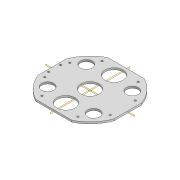
# Autodesk Inventor part: Drone_plate_3
Saved by Autodesk Inventor 2022 (Build 260153000, 153)
## iProperties
Created: 2022-04-28
Part Number: Drone_plate_3
Material: Generic
Document SubType Name: Modeling
Designer: dell
Density: 1 g/cm^3
Appearance: Default
Mass: 28.3386 g
Surface Area: 222.49 cm^2
Volume: 28.3386 cm^3
Author: dell
Autodesk Inventor part; units mm, degrees
ref_plane "XZ Plane" through (0, 0, 0) normal (0, 1, 0) x (-1, 0, 0)
ref_plane "XY Plane" through (0, 0, 0) normal (0, 0, 1) x (1, 0, 0)
sketch "Sketch1" plane through (0, 0, 0) normal (0, 1, 0) x (-1, 0, 0)
  line L0 (0, 0) -> (60, 0)
  line L1 (60, 0) -> (60, -120)
  line L2 (60, -120) -> (0, -120)
  line L3 (0, -120) -> (0, 0)
  line L4 (60, 0) -> (0, -120) construction
  line L5 (60, -120) -> (0, 0) construction
  circle A0 centre (30, -60) radius 67.082
  line L6 (30, -120) -> (30, 7.082) construction
  line L7 (60, -60) -> (0, -60)
  line L8 (30, -60) -> (81.3878, -103.1195) construction
  line L9 (41.76, -45.985) -> (17.4815, -74.919) construction
  line L10 (-33, -36.9566) -> (-33, -83.0434)
  line L11 (93, -36.9566) -> (93, -83.0434)
  circle A1 centre (60, -110) radius 1.5
  circle A2 centre (70, -60) radius 12.5
  circle A3 centre (30, -100) radius 15
  circle A4 centre (84.4498, -80.8618) radius 1.5
  circle A5 centre (68.3022, -92.1394) radius 10
  circle A6 centre (30, -60) radius 15
  point P0 (60, -120)
  point P1 (60, 0)
  dimension "d0" = 120
  dimension "d25" = 60
  dimension "d27" = 50
  dimension "d38" = 63
  dimension "d39" = 63
  dimension "d50" = 3
  dimension "d51" = 10
  dimension "d52" = 25
  dimension "d53" = 40
  dimension "d54" = 30
  dimension "d55" = 40
  dimension "d56" = 20
  dimension "d57" = 50
  dimension "d58" = 30
  constraints: 24 end point, 6 centre point, 6 midpoint, 4 point on line, 3 parallel, 3 perpendicular, 2 coincident, 1 horizontal, 1 horizontal alignment, 1 symmetric about line, 1 vertical, 10 other
  measures "d0" distance of L2.end L0.start
  measures "d25" distance between parallel lines of L1 L3
  measures "d27" angle of L6 L8
  measures "d38" distance from line of point (30, -60) L10
  measures "d39" distance from line of point (30, -60) L11
  measures "d50" diameter of A1
  measures "d51" distance of L1.end A1.centre
  measures "d52" diameter of A2
  measures "d53" distance of L8.start A2.centre
  measures "d54" diameter of A3
  measures "d55" distance of L8.start A3.centre
  measures "d56" diameter of A5
  measures "d57" distance of point (30, -60) A5.centre
  measures "d58" diameter of A6
extrude "Extrusion1" add sketch "Sketch1" along normal blind 3 contours L0 L1 A2 L7 A6 L3 | L3 A0 L10 | A0 L11 L1 A1 A5 A2 | L7 A6 A2 L1 A5 A1 L2 L3 | A2 L1 | L1 L7 A2 | A6 L7 | L7 A6 | L1 A2 L7 | A1 L1 | L1 A1 | A5 L1 | L1 A5 | A3 | A4
extrude "Extrusion3" cut sketch "Sketch1" along normal blind 10 contours A6 L7 | L7 A6 | A1 L1 | L1 A1 | A5 L1 | L1 A5 | A3 | A4
ref_plane "Work Plane5" through (-60, 0, -60) normal (0, 0, 1) x (1, 0, 0)
ref_plane "Work Plane6" through (-30, 0, 0) normal (1, 0, 0) x (0, 1, 0)
mirror "Mirror3" about plane through (-60, 0, -60) normal (0, 0, 1) of "Extrusion3"
mirror "Mirror4" about plane through (-30, 0, 0) normal (1, 0, 0) of "Extrusion3", "Mirror3"
sketch "Sketch10" plane through (0, 3, 0) normal (0, 1, 0) x (1, 0, 0)
  circle A0 centre (24.4498, 39.1382) radius 1.5 projected
  circle A1 centre (8.3022, 27.8606) radius 10 projected
  circle A2 centre (0, 10) radius 1.5 projected
  circle A3 centre (24.4498, 80.8618) radius 1.5 projected
  circle A4 centre (8.3022, 92.1394) radius 10 projected
  circle A5 centre (0, 110) radius 1.5 projected
  circle A6 centre (-84.4498, 39.1382) radius 1.5 projected
  circle A7 centre (-68.3022, 27.8606) radius 10 projected
  circle A8 centre (-60, 10) radius 1.5 projected
  circle A9 centre (-30, 20) radius 15 projected
  circle A10 centre (-84.4498, 80.8618) radius 1.5 projected
  circle A11 centre (-68.3022, 92.1394) radius 10 projected
  circle A12 centre (-60, 110) radius 1.5 projected
  circle A13 centre (-30, 100) radius 15 projected
  circle A14 centre (-30, 60) radius 15 projected
  line L0 (0, 120) -> (-60, 120) projected
  arc A15 (-60, 120) -> (-93, 83.0434) centre (-30, 60) ccw projected
  line L1 (-93, 83.0434) -> (-93, 36.9566) projected
  arc A16 (-93, 36.9566) -> (-60, 0) centre (-30, 60) ccw projected
  line L2 (-60, 0) -> (0, 0) projected
  arc A17 (0, 0) -> (33, 36.9566) centre (-30, 60) ccw projected
  line L3 (33, 36.9566) -> (33, 83.0434) projected
  arc A18 (33, 83.0434) -> (0, 120) centre (-30, 60) ccw projected
sketch "Sketch14" plane through (0, 3, 0) normal (0, 1, 0) x (1, 0, 0)
  circle A0 centre (-89, 70) radius 1.5
  circle A1 centre (-89, 50) radius 1.5
  line L0 (-93, 83.0434) -> (-93, 36.9566) projected
  line L1 (63.1517, 60) -> (-123.1517, 60) projected
  point P0 (0, 0)
  dimension "d75" = 3
  dimension "d76" = 3
  dimension "d77" = 4
  dimension "d78" = 4
  dimension "d79" = 10
  dimension "d80" = 10
  constraints: 2 centre point
  measures "d75" diameter of A0
  measures "d76" diameter of A1
  measures "d77" distance from line of L0 A1.centre
  measures "d78" distance from line of L0 A0.centre
  measures "d79" distance from line of L1 A0.centre
  measures "d80" distance from line of A1.centre L1
extrude "Extrusion6" cut sketch "Sketch14" against normal blind 10
body "Solid1"
